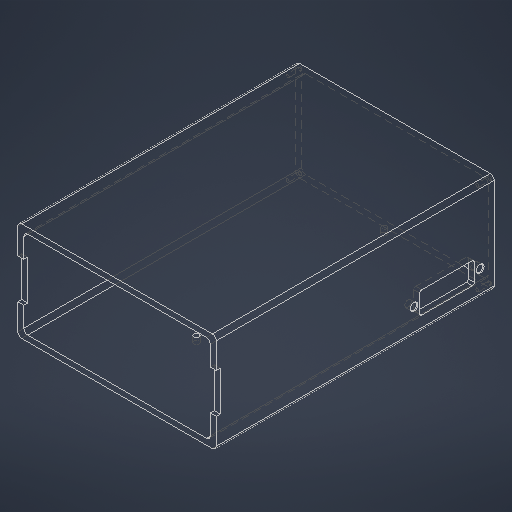
# Autodesk Inventor part: obudowa
Saved by Autodesk Inventor 2026.1 (Build 301233020, 233B)
## iProperties
Created: 2026-03-16
Part Number: obudowa
Material: Generic
Document SubType Name: Modeling
Designer: Jan
Density: 1 g/cm^3
Appearance: Default
Finish3_Appearance: Aluminum - Dark
Finish3_Area: 81068.516 mm^2
Author: Jan
Autodesk Inventor part; units mm, degrees
ref_plane "YZ Plane" through (0, 0, 0) normal (1, 0, 0) x (0, 1, 0)
ref_plane "XZ Plane" through (0, 0, 0) normal (0, 1, 0) x (-1, 0, 0)
ref_plane "XY Plane" through (0, 0, 0) normal (0, 0, 1) x (1, 0, 0)
sketch "Sketch1" plane through (0, 0, 0) normal (0, 0, 1) x (1, 0, 0)
  line L0 (2, 0) -> (92, 0)
  line L1 (94, 2) -> (94, 42)
  line L2 (92, 44) -> (2, 44)
  line L3 (0, 42) -> (0, 2)
  line L4 (-1, 47) -> (95, 47)
  line L5 (97, 45) -> (97, -1)
  line L6 (95, -3) -> (-1, -3)
  line L7 (-3, -1) -> (-3, 45)
  arc A0 (2, 44) -> (0, 42) centre (2, 42) ccw
  arc A1 (0, 2) -> (2, 0) centre (2, 2) ccw
  arc A2 (92, 0) -> (94, 2) centre (92, 2) ccw
  arc A3 (94, 42) -> (92, 44) centre (92, 42) ccw
  arc A4 (-3, -1) -> (-1, -3) centre (-1, -1) ccw
  arc A5 (-1, 47) -> (-3, 45) centre (-1, 45) ccw
  arc A6 (97, 45) -> (95, 47) centre (95, 45) ccw
  arc A7 (95, -3) -> (97, -1) centre (95, -1) ccw
  point P0 (0, 0)
  point P1 (94, 44)
  point P2 (94, 0)
  point P3 (0, 44)
  point P4 (97, -3)
  point P5 (97, 47)
  point P6 (-3, -3)
  dimension "d0" = 94
  dimension "d1" = 44
  dimension "d2" = 100
  dimension "d3" = 50
  dimension "d4" = 3
  dimension "d5" = 3
  dimension "d6" = 2
  dimension "d9" = 2
  constraints: 16 end point, 16 point on circle, 16 tangent, 14 point on line, 8 centre point, 6 equal radius, 4 parallel, 2 horizontal, 2 perpendicular
  measures "d0" distance of point (0, 44) point (94, 44)
  measures "d1" distance of point (94, 44) point (94, 0)
  measures "d2" distance of point (97, -3) point (-3, -3)
  measures "d3" distance of point (97, 47) point (97, -3)
  measures "d4" distance between parallel lines of L4 L2
  measures "d5" distance between parallel lines of L7 L3
  measures "d6" radius of A0
  measures "d9" radius of A7
extrude "Extrusion1" add sketch "Sketch1" along normal blind 140
sketch "Sketch2" plane through (0, 0, 140) normal (0, 0, 1) x (1, 0, 0)
  line L0 (-3, 45) -> (-3, -1) projected
  line L1 (97, -1) -> (97, 45) projected
  line L2 (-3, 32) -> (97, 32)
  line L3 (97, 32) -> (97, 12)
  line L4 (97, 12) -> (-3, 12)
  line L5 (-3, 12) -> (-3, 32)
  line L6 (-1, -3) -> (95, -3) projected
  line L7 (95, 47) -> (-1, 47) projected
  point P0 (0, 0)
  point P1 (-3, 12)
  dimension "d10" = 20
  dimension "d11" = 15
  dimension "d12" = 50
  constraints: 8 end point, 2 parallel, 2 point on line, 1 horizontal, 1 perpendicular
  measures "d10" distance between parallel lines of L2 L4
  measures "d11" distance between parallel lines of L4 L6
  measures "d12" distance between parallel lines of L7 L6
extrude "Extrusion2" cut sketch "Sketch2" against normal blind 2
sketch "Sketch3" plane through (97, -1, 0) normal (1, 0, 0) x (0, 0, -1)
  line L0 (-11, 5.5) -> (-36.5, 5.5)
  line L1 (-37.5, 6.5) -> (-37.5, 15.5)
  line L2 (-36.5, 16.5) -> (-11, 16.5)
  line L3 (-10, 15.5) -> (-10, 6.5)
  line L4 (0, -2) -> (-140, -2) projected
  line L5 (0, 48) -> (-140, 48) projected
  line L6 (0, 0) -> (0, 46) projected
  arc A0 (-11, 5.5) -> (-10, 6.5) centre (-11, 6.5) ccw
  arc A1 (-10, 15.5) -> (-11, 16.5) centre (-11, 15.5) ccw
  arc A2 (-37.5, 6.5) -> (-36.5, 5.5) centre (-36.5, 6.5) ccw
  arc A3 (-36.5, 16.5) -> (-37.5, 15.5) centre (-36.5, 15.5) ccw
  circle A4 centre (-7.09, 11) radius 1.5
  circle A5 centre (-40.41, 11) radius 1.5
  line L7 (-23.75, 5.5) -> (-23.75, 19.7829) construction
  point P0 (0, 1)
  point P1 (-37.5, 16.5)
  point P2 (-37.5, 5.5)
  point P3 (-10, 16.5)
  dimension "d15" = 27.5
  dimension "d16" = 11
  dimension "d17" = 50
  dimension "d18" = 31.5
  dimension "d19" = 10
  dimension "d20" = 1
  dimension "d21" = 3
  dimension "d22" = 3
  dimension "d23" = 16.66
  dimension "d24" = 16.66
  constraints: 10 end point, 8 point on circle, 8 tangent, 6 centre point, 6 point on line, 3 equal radius, 2 parallel, 1 horizontal, 1 midpoint, 1 perpendicular, 1 vertical
  measures "d15" distance of point (-37.5, 16.5) point (-10, 16.5)
  measures "d16" distance of point (-37.5, 5.5) point (-37.5, 16.5)
  measures "d17" distance between parallel lines of L4 L5
  measures "d18" distance from line of point (-10, 16.5) L5
  measures "d19" distance between parallel lines of L6 L3
  measures "d20" radius of A0
  measures "d21" diameter of A4
  measures "d22" diameter of A5
  measures "d23" distance from line of L7 A4.centre
  measures "d24" distance from line of A5.centre L7
extrude "Extrusion3" cut sketch "Sketch3" against normal blind 10 contours L0 A2 L1 A3 L2 A1 L3 A0
hole "Hole1" at (97, 10, 7.09) at (97, 10, 40.41) direction (-1, 0, 0) diameter 3.4 depth 8.8 tip angle 118 clearance for "Countersunk Flat Head Screw ISO 2009/7046" size "M3" standard "ISO"
chamfer "Chamfer1" distance 0.3 angle 45 2 edges at (97, 10, 8.79) (97, 10, 42.11)
sketch "Sketch5" plane through (-1, -3, 0) normal (0, -1, 0) x (1, 0, 0)
  circle A0 centre (45.75, 3.13) radius 1.5
  circle A1 centre (45.75, 97.75) radius 1.5
  line L0 (98, 0) -> (98, 140) projected
  line L1 (0, 0) -> (96, 0) projected
  point P0 (1, 0)
  dimension "d49" = 3
  dimension "d50" = 3
  dimension "d51" = 94.62
  dimension "d52" = 52.25
  dimension "d53" = 3.13
  constraints: 2 centre point, 1 vertical alignment
  measures "d49" diameter of A0
  measures "d50" diameter of A1
  measures "d51" distance of A0.centre A1.centre
  measures "d52" distance from line of A0.centre L0
  measures "d53" distance from line of L1 A0.centre
hole "Hole3" at (44.75, -3, 3.13) at (44.75, -3, 97.75) direction (0, 1, 0) diameter 2.6416 depth 10.979 tip angle 118 thread size "6-32 UNC" class "2B" standard "ANSI Unified Screw Threads"
sketch "Sketch6" plane through (0, 0, 0) normal (0, 0, -1) x (-1, 0, 0)
  circle A0 centre (0.8, -0.8) radius 1
  line L0 (1, -3) -> (-95, -3) construction
  line L1 (-47, -3) -> (-47, -11.0585) construction
  line L2 (3, 45) -> (3, -1) construction
  line L3 (3, 22) -> (17.9543, 22) construction
  circle A1 centre (0.8, 44.8) radius 1
  line L4 (-47, 47) -> (-47, 55.0585) construction
  circle A2 centre (-94.8, -0.8) radius 1
  circle A3 centre (-94.8, 44.8) radius 1
  point P0 (0, 0)
  point P1 (-94, 0)
  point P2 (-97, 45)
  point P3 (-97, -1)
  dimension "d61" = 2
  dimension "d62" = 2.2
  dimension "d63" = 2.2
  constraints: 8 symmetric about line, 6 end point, 4 centre point, 2 midpoint, 1 horizontal, 1 vertical, 3 other
  measures "d61" diameter of A0
  measures "d62" distance from line of L0 A0.centre
  measures "d63" distance from line of L2 A0.centre
hole "Hole4" at (-0.8, -0.8, 0) at (-0.8, 44.8, 0) at (94.8, 44.8, 0) at (94.8, -0.8, 0) direction (0, 0, 1) diameter 1.567 depth 6.3 tip angle 118 thread size "M2x0.4" class "6H" standard "ISO Metric profile"
chamfer "Chamfer2" distance 0.2 angle 45 4 edges at (-0.8, -1.5835, 0) (-0.8, 44.0165, 0) (94.8, 44.0165, 0) (94.8, -1.5835, 0)
equation "\"d24\" = d23"
body "Solid1"
